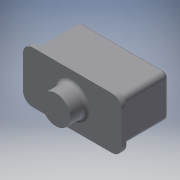
# Autodesk Inventor part: Button
Saved by Autodesk Inventor 2017 (Build 210142000, 142)
## iProperties
Created: 2019-05-31
Part Number: Button
Material: Generic
Document SubType Name: Modeling
Designer: Mitch
Density: 1 g/cm^3
Appearance: Default
Author: Mitch
Autodesk Inventor part; units mm, degrees
ref_plane "YZ Plane" through (0, 0, 0) normal (1, 0, 0) x (0, 1, 0)
ref_plane "XZ Plane" through (0, 0, 0) normal (0, 1, 0) x (-1, 0, 0)
ref_plane "XY Plane" through (0, 0, 0) normal (0, 0, 1) x (1, 0, 0)
sketch "Sketch1" plane through (0, 0, 0) normal (0, 0, 1) x (1, 0, 0)
  spline S0 degree 3 poles (-2.1619, 2.5084) (-2.0637, 2.5491) (-1.9573, 2.5689) (-1.7578, 2.5689) (-1.6511, 2.5489) (-1.4547, 2.4672) (-1.365, 2.4055) (-1.2248, 2.2641) (-1.1644, 2.1755) (-1.084, 1.9808) (-1.0641, 1.8748) (-1.0641, 1.7752) (-1.0641, 1.6756) (-1.084, 1.5695) (-1.1242, 1.4722) knots 0 0 0 0 0.167835 0.167835 0.336607 0.336607 0.505378 0.505378 0.670252 0.670252 0.835126 0.835126 0.835126 1 1 1 1
  line L0 (-1.8578, 2.5689) -> (-10.4303, 2.5689)
  spline S1 degree 3 poles (-11.164, 1.4722) (-11.2042, 1.5695) (-11.2241, 1.6756) (-11.2241, 1.8748) (-11.2042, 1.9808) (-11.1238, 2.1755) (-11.0633, 2.2641) (-10.9232, 2.4055) (-10.8335, 2.4672) (-10.6371, 2.5489) (-10.5304, 2.5689) (-10.3308, 2.5689) (-10.2244, 2.5491) (-10.1263, 2.5084) knots 0 0 0 0 0.164863 0.164863 0.329726 0.329726 0.49459 0.49459 0.663373 0.663373 0.832156 0.832156 1 1 1 1
  line L1 (-11.2241, 1.7752) -> (-11.2241, -1.7137)
  spline S2 degree 3 poles (-10.1263, -2.4469) (-10.2244, -2.4876) (-10.3308, -2.5075) (-10.5304, -2.5075) (-10.6371, -2.4874) (-10.8335, -2.4057) (-10.9232, -2.344) (-11.0633, -2.2026) (-11.1238, -2.114) (-11.2042, -1.9194) (-11.2241, -1.8133) (-11.2241, -1.6141) (-11.2042, -1.5081) (-11.164, -1.4107) knots 0 0 0 0 0.167844 0.167844 0.336627 0.336627 0.50541 0.50541 0.670274 0.670274 0.835137 0.835137 1 1 1 1
  line L2 (-10.4303, -2.5075) -> (-1.8578, -2.5075)
  spline S3 degree 3 poles (-1.1242, -1.4107) (-1.084, -1.5081) (-1.0641, -1.6141) (-1.0641, -1.7137) (-1.0641, -1.8133) (-1.084, -1.9194) (-1.1644, -2.114) (-1.2248, -2.2026) (-1.365, -2.344) (-1.4547, -2.4057) (-1.6511, -2.4874) (-1.7578, -2.5075) (-1.9573, -2.5075) (-2.0637, -2.4876) (-2.1619, -2.4469) knots 0 0 0 0 0.164874 0.164874 0.164874 0.329748 0.329748 0.494622 0.494622 0.663393 0.663393 0.832165 0.832165 1 1 1 1
  line L3 (-1.0641, -1.7137) -> (-1.0641, 1.7752)
  line L4 (-10.4303, 2.3149) -> (-1.8578, 2.3149)
  line L5 (-1.3181, 1.7752) -> (-1.3181, -1.7137)
  line L6 (-1.8578, -2.2535) -> (-10.4303, -2.2535)
  line L7 (-10.9701, -1.7137) -> (-10.9701, 1.7752)
  spline S4 degree 5 poles (-1.8578, 2.3148) (-1.6882, 2.3149) (-1.5187, 2.2484) (-1.3846, 2.1143) (-1.3181, 1.9448) (-1.3182, 1.7752) knots 0 0 0 0 0 0 1 1 1 1 1 1
  spline S5 degree 5 poles (-1.3182, -1.7137) (-1.3181, -1.8833) (-1.3846, -2.0528) (-1.5187, -2.1869) (-1.6882, -2.2535) (-1.8578, -2.2533) knots 0 0 0 0 0 0 1 1 1 1 1 1
  spline S6 degree 5 poles (-10.4303, -2.2533) (-10.5999, -2.2535) (-10.7694, -2.1869) (-10.9035, -2.0528) (-10.9701, -1.8833) (-10.97, -1.7137) knots 0 0 0 0 0 0 1 1 1 1 1 1
  spline S7 degree 5 poles (-10.97, 1.7752) (-10.9701, 1.9448) (-10.9035, 2.1143) (-10.7694, 2.2484) (-10.5999, 2.3149) (-10.4303, 2.3148) knots 0 0 0 0 0 0 1 1 1 1 1 1
  point P0 (0, 0)
  dimension "d0" = 0.254
  constraints: 8 end point, 7 parallel, 12 other
  measures "d0" distance between parallel lines of L0 L4
extrude "Extrusion1" add sketch "Sketch1" against normal blind 5.08 contours L4 S4 L5 S5 L6 S6 L7 S7
sketch "Sketch2" plane through (0, 0, 0) normal (0, 0, 1) x (1, 0, 0)
  line L0 (-10.4303, 2.3149) -> (-1.8578, 2.3149) projected
  spline S0 degree 5 poles (-10.9701, 1.7752) (-10.9701, 1.9448) (-10.9035, 2.1143) (-10.7694, 2.2484) (-10.5999, 2.3149) (-10.4303, 2.3149) knots 0 0 0 0 0 0 1 1 1 1 1 1
  line L1 (-10.9701, -1.7137) -> (-10.9701, 1.7752) projected
  spline S1 degree 5 poles (-10.4303, -2.2535) (-10.5999, -2.2535) (-10.7694, -2.1869) (-10.9035, -2.0528) (-10.9701, -1.8833) (-10.97, -1.7137) knots 0 0 0 0 0 0 1 1 1 1 1 1
  line L2 (-1.8578, -2.2535) -> (-10.4303, -2.2535) projected
  spline S2 degree 5 poles (-1.3181, -1.7137) (-1.3181, -1.8833) (-1.3846, -2.0528) (-1.5187, -2.1869) (-1.6882, -2.2535) (-1.8578, -2.2533) knots 0 0 0 0 0 0 1 1 1 1 1 1
  line L3 (-1.3181, 1.7752) -> (-1.3181, -1.7137) projected
  spline S3 degree 5 poles (-1.8578, 2.3149) (-1.6882, 2.3149) (-1.5187, 2.2484) (-1.3846, 2.1143) (-1.3181, 1.9448) (-1.3182, 1.7752) knots 0 0 0 0 0 0 1 1 1 1 1 1
  line L4 (-1.8578, 2.8229) -> (-10.4303, 2.8229)
  line L5 (-11.4781, 1.7752) -> (-11.4781, -1.7137)
  line L6 (-10.4303, -2.7615) -> (-1.8578, -2.7615)
  line L7 (-0.8101, -1.7137) -> (-0.8101, 1.7752)
  spline S4 degree 5 poles (-10.4303, 2.8229) (-10.7594, 2.8229) (-11.0889, 2.6938) (-11.349, 2.4338) (-11.4781, 2.1043) (-11.4781, 1.7752) knots 0 0 0 0 0 0 1 1 1 1 1 1
  spline S5 degree 5 poles (-11.478, -1.7133) (-11.4782, -2.0425) (-11.3491, -2.3721) (-11.089, -2.6323) (-10.7595, -2.7614) (-10.4303, -2.7615) knots 0 0 0 0 0 0 1 1 1 1 1 1
  spline S6 degree 5 poles (-1.8582, -2.7613) (-1.529, -2.7616) (-1.1994, -2.6325) (-0.9392, -2.3724) (-0.8101, -2.0429) (-0.8101, -1.7137) knots 0 0 0 0 0 0 1 1 1 1 1 1
  spline S7 degree 5 poles (-0.8102, 1.7748) (-0.81, 2.104) (-0.939, 2.4336) (-1.1991, 2.6938) (-1.5287, 2.8229) (-1.8578, 2.8229) knots 0 0 0 0 0 0 1 1 1 1 1 1
  point P0 (0, 0)
  dimension "d3" = 0.508
  constraints: 8 end point, 7 parallel, 16 other
  measures "d3" distance between parallel lines of L0 L4
extrude "Extrusion2" add sketch "Sketch2" along normal blind 0.508 contours L0 S3 L3 S2 L2 S1 L1 S0 | S7 L7 S6 L6 S5 L5 S4 L4
fillet "Fillet1" radius 0.381 16 edges at (-1.4763, 2.1567, -5.08) (-1.3181, 0.0307, -5.08) (-1.4763, -2.0952, -5.08) (-6.1441, -2.2534, -5.08) (-10.8119, -2.0953, -5.08) (-10.97, 0.0307, -5.08) (-10.8119, 2.1567, -5.08) (-6.1441, 2.3149, -5.08) (-1.4763, -2.0952, 0) (-6.1441, -2.2534, 0) (-10.8119, -2.0953, 0) (-10.97, 0.0307, 0) (-10.8119, 2.1567, 0) (-6.1441, 2.3149, 0) (-1.4763, 2.1567, 0) (-1.3181, 0.0307, 0)
sketch "Sketch3" plane through (0, 0, 0.508) normal (0, 0, 1) x (1, 0, 0)
  circle A0 centre (-6.1441, 0.0325) radius 1.5475 projected
  point P0 (0, 0)
extrude "Extrusion3" add sketch "Sketch3" along normal blind 1.778
fillet "Fillet2" radius 0.381 1 edges at (-7.6916, 0.0325, 0.508)
body "Solid1"
